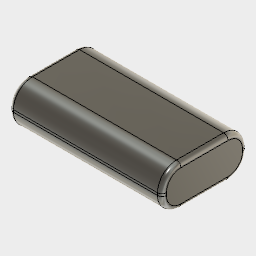
354 4400mah battery (Autodesk Fusion 360 design; units mm, degrees)
Autodesk Fusion 360 part; units mm, degrees
sketch "Sketch1" plane through (0, 0, 0) normal (0, 0, 1) x (1, 0, 0)
  line L0 (0, 0) -> (68.58, 0)
  line L1 (68.58, 0) -> (68.58, 38.1)
  line L2 (68.58, 38.1) -> (0, 38.1)
  line L3 (0, 38.1) -> (0, 0)
  dimension "d1" = 68.58
  dimension "d2" = 38.1
  measures "d1" distance of L0.start L0.end
  measures "d2" distance of L0.start L2.end
extrude "Extrude1" add sketch "Sketch1" along normal blind 18.034
fillet "Fillet1" radius 8.5 4 edges at (34.29, 38.1, 0) (34.29, 38.1, 18.034) (34.29, 0, 0) (34.29, 0, 18.034)
fillet "Fillet2" radius 2 16 edges at (0, 0, 9.017) (0, 2.4896, 2.4896) (0, 19.05, 0) (0, 35.6104, 2.4896) (0, 38.1, 9.017) (0, 35.6104, 15.5444) (0, 19.05, 18.034) (0, 2.4896, 15.5444) (68.58, 38.1, 9.017) (68.58, 35.6104, 2.4896) (68.58, 19.05, 0) (68.58, 2.4896, 2.4896) (68.58, 0, 9.017) (68.58, 2.4896, 15.5444) (68.58, 19.05, 18.034) (68.58, 35.6104, 15.5444)
